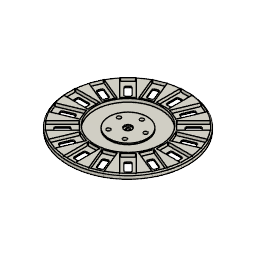
Brodie Rotor (Autodesk Fusion 360 design; units mm, degrees)
Autodesk Fusion 360 part; units mm, degrees
sketch "Sketch1" plane through (0, 0, 0) normal (0, 0, 1) x (1, 0, 0)
  circle A0 centre (0, 0) radius 26
  line L0 (-4.2, 27) -> (4.2, 27)
  line L1 (4.5, 27.3) -> (4.5, 45.7)
  line L2 (4.2, 46) -> (-4.2, 46)
  line L3 (-4.5, 45.7) -> (-4.5, 27.3)
  circle A1 centre (0, 0) radius 47
  line L4 (-4.5, 36.5) -> (4.5, 36.5) construction
  arc A2 (4.2, 27) -> (4.5, 27.3) centre (4.5, 27) ccw
  arc A3 (-4.5, 27.3) -> (-4.2, 27) centre (-4.5, 27) ccw
  arc A4 (-4.2, 46) -> (-4.5, 45.7) centre (-4.5, 46) ccw
  arc A5 (4.5, 45.7) -> (4.2, 46) centre (4.5, 46) ccw
  arc A6 (-13.3312, 43.9434) -> (-13.7231, 44.1057) centre (-13.446, 44.2205) ccw
  line L5 (-6.2898, 26.944) -> (-13.3312, 43.9434)
  line L6 (-13.7231, 44.1057) -> (-21.4837, 40.8912)
  arc A7 (-21.4837, 40.8912) -> (-21.6461, 40.4992) centre (-21.7609, 40.7764) ccw
  line L7 (-21.6461, 40.4992) -> (-14.6047, 23.4998)
  arc A8 (-14.6047, 23.4998) -> (-14.2127, 23.3375) centre (-14.4899, 23.2227) ccw
  line L8 (-14.2127, 23.3375) -> (-6.4522, 26.552)
  arc A9 (-6.4522, 26.552) -> (-6.2898, 26.944) centre (-6.175, 26.6668) ccw
  arc A10 (-29.1328, 35.4968) -> (-29.5571, 35.4968) centre (-29.3449, 35.7089) ccw
  line L9 (-16.122, 22.486) -> (-29.1328, 35.4968)
  line L10 (-29.5571, 35.4968) -> (-35.4968, 29.5571)
  arc A11 (-35.4968, 29.5571) -> (-35.4968, 29.1328) centre (-35.7089, 29.3449) ccw
  line L11 (-35.4968, 29.1328) -> (-22.486, 16.122)
  arc A12 (-22.486, 16.122) -> (-22.0617, 16.122) centre (-22.2739, 15.9099) ccw
  line L12 (-22.0617, 16.122) -> (-16.122, 22.0617)
  arc A13 (-16.122, 22.0617) -> (-16.122, 22.486) centre (-15.9099, 22.2739) ccw
  arc A14 (-40.4992, 21.6461) -> (-40.8912, 21.4837) centre (-40.7764, 21.7609) ccw
  line L13 (-23.4998, 14.6047) -> (-40.4992, 21.6461)
  line L14 (-40.8912, 21.4837) -> (-44.1057, 13.7231)
  arc A15 (-44.1057, 13.7231) -> (-43.9434, 13.3312) centre (-44.2205, 13.446) ccw
  line L15 (-43.9434, 13.3312) -> (-26.944, 6.2898)
  arc A16 (-26.944, 6.2898) -> (-26.552, 6.4522) centre (-26.6668, 6.175) ccw
  line L16 (-26.552, 6.4522) -> (-23.3375, 14.2127)
  arc A17 (-23.3375, 14.2127) -> (-23.4998, 14.6047) centre (-23.2227, 14.4899) ccw
  arc A18 (-45.7, 4.5) -> (-46, 4.2) centre (-46, 4.5) ccw
  line L17 (-27.3, 4.5) -> (-45.7, 4.5)
  line L18 (-46, 4.2) -> (-46, -4.2)
  arc A19 (-46, -4.2) -> (-45.7, -4.5) centre (-46, -4.5) ccw
  line L19 (-45.7, -4.5) -> (-27.3, -4.5)
  arc A20 (-27.3, -4.5) -> (-27, -4.2) centre (-27, -4.5) ccw
  line L20 (-27, -4.2) -> (-27, 4.2)
  arc A21 (-27, 4.2) -> (-27.3, 4.5) centre (-27, 4.5) ccw
  arc A22 (-43.9434, -13.3312) -> (-44.1057, -13.7231) centre (-44.2205, -13.446) ccw
  line L21 (-26.944, -6.2898) -> (-43.9434, -13.3312)
  line L22 (-44.1057, -13.7231) -> (-40.8912, -21.4837)
  arc A23 (-40.8912, -21.4837) -> (-40.4992, -21.6461) centre (-40.7764, -21.7609) ccw
  line L23 (-40.4992, -21.6461) -> (-23.4998, -14.6047)
  arc A24 (-23.4998, -14.6047) -> (-23.3375, -14.2127) centre (-23.2227, -14.4899) ccw
  line L24 (-23.3375, -14.2127) -> (-26.552, -6.4522)
  arc A25 (-26.552, -6.4522) -> (-26.944, -6.2898) centre (-26.6668, -6.175) ccw
  arc A26 (-35.4968, -29.1328) -> (-35.4968, -29.5571) centre (-35.7089, -29.3449) ccw
  line L25 (-22.486, -16.122) -> (-35.4968, -29.1328)
  line L26 (-35.4968, -29.5571) -> (-29.5571, -35.4968)
  arc A27 (-29.5571, -35.4968) -> (-29.1328, -35.4968) centre (-29.3449, -35.7089) ccw
  line L27 (-29.1328, -35.4968) -> (-16.122, -22.486)
  arc A28 (-16.122, -22.486) -> (-16.122, -22.0617) centre (-15.9099, -22.2739) ccw
  line L28 (-16.122, -22.0617) -> (-22.0617, -16.122)
  arc A29 (-22.0617, -16.122) -> (-22.486, -16.122) centre (-22.2739, -15.9099) ccw
  arc A30 (-21.6461, -40.4992) -> (-21.4837, -40.8912) centre (-21.7609, -40.7764) ccw
  line L29 (-14.6047, -23.4998) -> (-21.6461, -40.4992)
  line L30 (-21.4837, -40.8912) -> (-13.7231, -44.1057)
  arc A31 (-13.7231, -44.1057) -> (-13.3312, -43.9434) centre (-13.446, -44.2205) ccw
  line L31 (-13.3312, -43.9434) -> (-6.2898, -26.944)
  arc A32 (-6.2898, -26.944) -> (-6.4522, -26.552) centre (-6.175, -26.6668) ccw
  line L32 (-6.4522, -26.552) -> (-14.2127, -23.3375)
  arc A33 (-14.2127, -23.3375) -> (-14.6047, -23.4998) centre (-14.4899, -23.2227) ccw
  arc A34 (-4.5, -45.7) -> (-4.2, -46) centre (-4.5, -46) ccw
  line L33 (-4.5, -27.3) -> (-4.5, -45.7)
  line L34 (-4.2, -46) -> (4.2, -46)
  arc A35 (4.2, -46) -> (4.5, -45.7) centre (4.5, -46) ccw
  line L35 (4.5, -45.7) -> (4.5, -27.3)
  arc A36 (4.5, -27.3) -> (4.2, -27) centre (4.5, -27) ccw
  line L36 (4.2, -27) -> (-4.2, -27)
  arc A37 (-4.2, -27) -> (-4.5, -27.3) centre (-4.5, -27) ccw
  arc A38 (13.3312, -43.9434) -> (13.7231, -44.1057) centre (13.446, -44.2205) ccw
  line L37 (6.2898, -26.944) -> (13.3312, -43.9434)
  line L38 (13.7231, -44.1057) -> (21.4837, -40.8912)
  arc A39 (21.4837, -40.8912) -> (21.6461, -40.4992) centre (21.7609, -40.7764) ccw
  line L39 (21.6461, -40.4992) -> (14.6047, -23.4998)
  arc A40 (14.6047, -23.4998) -> (14.2127, -23.3375) centre (14.4899, -23.2227) ccw
  line L40 (14.2127, -23.3375) -> (6.4522, -26.552)
  arc A41 (6.4522, -26.552) -> (6.2898, -26.944) centre (6.175, -26.6668) ccw
  arc A42 (29.1328, -35.4968) -> (29.5571, -35.4968) centre (29.3449, -35.7089) ccw
  line L41 (16.122, -22.486) -> (29.1328, -35.4968)
  line L42 (29.5571, -35.4968) -> (35.4968, -29.5571)
  arc A43 (35.4968, -29.5571) -> (35.4968, -29.1328) centre (35.7089, -29.3449) ccw
  line L43 (35.4968, -29.1328) -> (22.486, -16.122)
  arc A44 (22.486, -16.122) -> (22.0617, -16.122) centre (22.2739, -15.9099) ccw
  line L44 (22.0617, -16.122) -> (16.122, -22.0617)
  arc A45 (16.122, -22.0617) -> (16.122, -22.486) centre (15.9099, -22.2739) ccw
  arc A46 (40.4992, -21.6461) -> (40.8912, -21.4837) centre (40.7764, -21.7609) ccw
  line L45 (23.4998, -14.6047) -> (40.4992, -21.6461)
  line L46 (40.8912, -21.4837) -> (44.1057, -13.7231)
  arc A47 (44.1057, -13.7231) -> (43.9434, -13.3312) centre (44.2205, -13.446) ccw
  line L47 (43.9434, -13.3312) -> (26.944, -6.2898)
  arc A48 (26.944, -6.2898) -> (26.552, -6.4522) centre (26.6668, -6.175) ccw
  line L48 (26.552, -6.4522) -> (23.3375, -14.2127)
  arc A49 (23.3375, -14.2127) -> (23.4998, -14.6047) centre (23.2227, -14.4899) ccw
  arc A50 (45.7, -4.5) -> (46, -4.2) centre (46, -4.5) ccw
  line L49 (27.3, -4.5) -> (45.7, -4.5)
  line L50 (46, -4.2) -> (46, 4.2)
  arc A51 (46, 4.2) -> (45.7, 4.5) centre (46, 4.5) ccw
  line L51 (45.7, 4.5) -> (27.3, 4.5)
  arc A52 (27.3, 4.5) -> (27, 4.2) centre (27, 4.5) ccw
  line L52 (27, 4.2) -> (27, -4.2)
  arc A53 (27, -4.2) -> (27.3, -4.5) centre (27, -4.5) ccw
  arc A54 (43.9434, 13.3312) -> (44.1057, 13.7231) centre (44.2205, 13.446) ccw
  line L53 (26.944, 6.2898) -> (43.9434, 13.3312)
  line L54 (44.1057, 13.7231) -> (40.8912, 21.4837)
  arc A55 (40.8912, 21.4837) -> (40.4992, 21.6461) centre (40.7764, 21.7609) ccw
  line L55 (40.4992, 21.6461) -> (23.4998, 14.6047)
  arc A56 (23.4998, 14.6047) -> (23.3375, 14.2127) centre (23.2227, 14.4899) ccw
  line L56 (23.3375, 14.2127) -> (26.552, 6.4522)
  arc A57 (26.552, 6.4522) -> (26.944, 6.2898) centre (26.6668, 6.175) ccw
  arc A58 (35.4968, 29.1328) -> (35.4968, 29.5571) centre (35.7089, 29.3449) ccw
  line L57 (22.486, 16.122) -> (35.4968, 29.1328)
  line L58 (35.4968, 29.5571) -> (29.5571, 35.4968)
  arc A59 (29.5571, 35.4968) -> (29.1328, 35.4968) centre (29.3449, 35.7089) ccw
  line L59 (29.1328, 35.4968) -> (16.122, 22.486)
  arc A60 (16.122, 22.486) -> (16.122, 22.0617) centre (15.9099, 22.2739) ccw
  line L60 (16.122, 22.0617) -> (22.0617, 16.122)
  arc A61 (22.0617, 16.122) -> (22.486, 16.122) centre (22.2739, 15.9099) ccw
  arc A62 (21.6461, 40.4992) -> (21.4837, 40.8912) centre (21.7609, 40.7764) ccw
  line L61 (14.6047, 23.4998) -> (21.6461, 40.4992)
  line L62 (21.4837, 40.8912) -> (13.7231, 44.1057)
  arc A63 (13.7231, 44.1057) -> (13.3312, 43.9434) centre (13.446, 44.2205) ccw
  line L63 (13.3312, 43.9434) -> (6.2898, 26.944)
  arc A64 (6.2898, 26.944) -> (6.4522, 26.552) centre (6.175, 26.6668) ccw
  line L64 (6.4522, 26.552) -> (14.2127, 23.3375)
  arc A65 (14.2127, 23.3375) -> (14.6047, 23.4998) centre (14.4899, 23.2227) ccw
  dimension "d1" = 52
  dimension "d6" = 94
  dimension "d7" = 0.6
  dimension "d8" = 0.6
  dimension "d10" = 360
  constraint coincident A0.centre A1.centre
  constraint horizontal L0
  constraint vertical L1
  constraint horizontal L2
  constraint vertical L3
  constraint concentric A0 A1
  constraint symmetric L4 A3 A4
  constraint symmetric L4 A2 A5
  constraint coincident L1 L4.end
  constraint coincident L3 L4.start
  measures "d1" diameter of A0
  measures "d6" diameter of A1
  measures "d7" diameter of A4
  measures "d8" diameter of A5
extrude "Extrude1" add sketch "Sketch1" along normal blind 2.5
sketch "Sketch2" plane through (0, 0, 0) normal (0, 0, 1) x (1, 0, 0)
  circle A0 centre (0, 0) radius 47
  dimension "d13" = 94
  constraint coincident A0.centre origin
  measures "d13" diameter of A0
extrude "Extrude2" add sketch "Sketch2" against normal blind 1
move_body "Move1" bodies 1 to x (1, 0, 0) y (0, 1, 0) z (0, 0, 1) at (0, 0, 1)
sketch "Sketch3" plane through (0, 0, 1) normal (0, 0, 1) x (-1, 0, 0)
  circle A0 centre (0, 0) radius 26
  circle A1 centre (0, 0) radius 15
  dimension "d16" = 30
  constraint coincident A0.centre A1.centre
  measures "d16" diameter of A1
extrude "Extrude3" add sketch "Sketch3" along normal blind 1 contours A1
sketch "Sketch4" plane through (0, 0, 2) normal (0, 0, 1) x (-1, 0, 0)
  circle A0 centre (0, 0) radius 15
  circle A1 centre (0, 0) radius 3
  circle A2 centre (0, -11) radius 1.5
  circle A3 centre (10.4616, -3.3992) radius 1.5
  circle A4 centre (6.4656, 8.8992) radius 1.5
  circle A5 centre (-6.4656, 8.8992) radius 1.5
  circle A6 centre (-10.4616, -3.3992) radius 1.5
  dimension "d19" = 3
  dimension "d21" = 360
  constraint coincident A0.centre A1.centre
  measures "d19" diameter of A2
extrude "Extrude4" cut sketch "Sketch4" against normal blind 10 contours A2 | A3 | A4 | A5 | A6
extrude "Extrude5" add sketch "Sketch4" along normal blind 1 contours A1
sketch "Sketch5" plane through (0, 0, 3) normal (0, 0, 1) x (-1, 0, 0)
  circle A0 centre (0, 0) radius 3
  circle A1 centre (0, 0) radius 1.5
  dimension "d26" = 3
  constraint coincident A0.centre A1.centre
  measures "d26" diameter of A1
extrude "Extrude6" cut sketch "Sketch5" against normal blind 10 contours A1
extrude "Extrude7" cut 1 faces at (-2.4832, 0.2236, 3) along direction (0, 0, -1) blind 2
sketch "Sketch6" plane through (0, 0, 0) normal (0, 0, -1) x (1, 0, 0)
  circle A0 centre (0, 0) radius 1.5
  circle A1 centre (-6.4656, 8.8992) radius 1.5
  circle A2 centre (-10.4616, -3.3992) radius 1.5
  circle A3 centre (6.4656, 8.8992) radius 1.5
  circle A4 centre (0, -11) radius 1.5
  circle A5 centre (10.4616, -3.3992) radius 1.5
  circle A6 centre (0, 0) radius 47
  line L0 (-1.25, -31.75) -> (1.25, -31.75)
  line L1 (2.25, -32.75) -> (2.25, -40.25)
  line L2 (1.25, -41.25) -> (-1.25, -41.25)
  line L3 (-2.25, -40.25) -> (-2.25, -32.75)
  arc A7 (1.25, -41.25) -> (2.25, -40.25) centre (1.25, -40.25) ccw
  arc A8 (-2.25, -40.25) -> (-1.25, -41.25) centre (-1.25, -40.25) ccw
  arc A9 (-1.25, -31.75) -> (-2.25, -32.75) centre (-1.25, -32.75) ccw
  arc A10 (2.25, -32.75) -> (1.25, -31.75) centre (1.25, -32.75) ccw
  line L4 (2.25, -31.75) -> (2.0564, -32.1587) construction
  line L5 (-2.0564, -40.8413) -> (-2.25, -41.25) construction
  line L6 (-2.25, -31.75) -> (-2.0564, -32.1587) construction
  line L7 (2.0564, -40.8413) -> (2.25, -41.25) construction
  line L8 (13.3243, -38.0472) -> (10.4542, -31.1181)
  arc A11 (10.9953, -29.8115) -> (10.4542, -31.1181) centre (11.378, -30.7354) ccw
  arc A12 (14.6116, -29.396) -> (13.305, -28.8548) centre (13.6877, -29.7787) ccw
  line L9 (10.9953, -29.8115) -> (13.305, -28.8548)
  line L10 (14.6116, -29.396) -> (17.4817, -36.3251)
  arc A13 (16.9405, -37.6317) -> (17.4817, -36.3251) centre (16.5579, -36.7078) ccw
  line L11 (16.9405, -37.6317) -> (14.6308, -38.5884)
  arc A14 (13.3243, -38.0472) -> (14.6308, -38.5884) centre (14.2482, -37.6645) ccw
  line L12 (26.8701, -30.052) -> (21.5668, -24.7487)
  arc A15 (21.5668, -23.3345) -> (21.5668, -24.7487) centre (22.2739, -24.0416) ccw
  arc A16 (24.7487, -21.5668) -> (23.3345, -21.5668) centre (24.0416, -22.2739) ccw
  line L13 (21.5668, -23.3345) -> (23.3345, -21.5668)
  line L14 (24.7487, -21.5668) -> (30.052, -26.8701)
  arc A17 (30.052, -28.2843) -> (30.052, -26.8701) centre (29.3449, -27.5772) ccw
  line L15 (30.052, -28.2843) -> (28.2843, -30.052)
  arc A18 (26.8701, -30.052) -> (28.2843, -30.052) centre (27.5772, -29.3449) ccw
  line L16 (36.3251, -17.4817) -> (29.396, -14.6116)
  arc A19 (28.8548, -13.305) -> (29.396, -14.6116) centre (29.7787, -13.6877) ccw
  arc A20 (31.1181, -10.4542) -> (29.8115, -10.9953) centre (30.7354, -11.378) ccw
  line L17 (28.8548, -13.305) -> (29.8115, -10.9953)
  line L18 (31.1181, -10.4542) -> (38.0472, -13.3243)
  arc A21 (38.5884, -14.6308) -> (38.0472, -13.3243) centre (37.6645, -14.2482) ccw
  line L19 (38.5884, -14.6308) -> (37.6317, -16.9405)
  arc A22 (36.3251, -17.4817) -> (37.6317, -16.9405) centre (36.7078, -16.5579) ccw
  line L20 (40.25, -2.25) -> (32.75, -2.25)
  arc A23 (31.75, -1.25) -> (32.75, -2.25) centre (32.75, -1.25) ccw
  arc A24 (32.75, 2.25) -> (31.75, 1.25) centre (32.75, 1.25) ccw
  line L21 (31.75, -1.25) -> (31.75, 1.25)
  line L22 (32.75, 2.25) -> (40.25, 2.25)
  arc A25 (41.25, 1.25) -> (40.25, 2.25) centre (40.25, 1.25) ccw
  line L23 (41.25, 1.25) -> (41.25, -1.25)
  arc A26 (40.25, -2.25) -> (41.25, -1.25) centre (40.25, -1.25) ccw
  line L24 (38.0472, 13.3243) -> (31.1181, 10.4542)
  arc A27 (29.8115, 10.9953) -> (31.1181, 10.4542) centre (30.7354, 11.378) ccw
  arc A28 (29.396, 14.6116) -> (28.8548, 13.305) centre (29.7787, 13.6877) ccw
  line L25 (29.8115, 10.9953) -> (28.8548, 13.305)
  line L26 (29.396, 14.6116) -> (36.3251, 17.4817)
  arc A29 (37.6317, 16.9405) -> (36.3251, 17.4817) centre (36.7078, 16.5579) ccw
  line L27 (37.6317, 16.9405) -> (38.5884, 14.6308)
  arc A30 (38.0472, 13.3243) -> (38.5884, 14.6308) centre (37.6645, 14.2482) ccw
  line L28 (30.052, 26.8701) -> (24.7487, 21.5668)
  arc A31 (23.3345, 21.5668) -> (24.7487, 21.5668) centre (24.0416, 22.2739) ccw
  arc A32 (21.5668, 24.7487) -> (21.5668, 23.3345) centre (22.2739, 24.0416) ccw
  line L29 (23.3345, 21.5668) -> (21.5668, 23.3345)
  line L30 (21.5668, 24.7487) -> (26.8701, 30.052)
  arc A33 (28.2843, 30.052) -> (26.8701, 30.052) centre (27.5772, 29.3449) ccw
  line L31 (28.2843, 30.052) -> (30.052, 28.2843)
  arc A34 (30.052, 26.8701) -> (30.052, 28.2843) centre (29.3449, 27.5772) ccw
  line L32 (17.4817, 36.3251) -> (14.6116, 29.396)
  arc A35 (13.305, 28.8548) -> (14.6116, 29.396) centre (13.6877, 29.7787) ccw
  arc A36 (10.4542, 31.1181) -> (10.9953, 29.8115) centre (11.378, 30.7354) ccw
  line L33 (13.305, 28.8548) -> (10.9953, 29.8115)
  line L34 (10.4542, 31.1181) -> (13.3243, 38.0472)
  arc A37 (14.6308, 38.5884) -> (13.3243, 38.0472) centre (14.2482, 37.6645) ccw
  line L35 (14.6308, 38.5884) -> (16.9405, 37.6317)
  arc A38 (17.4817, 36.3251) -> (16.9405, 37.6317) centre (16.5579, 36.7078) ccw
  line L36 (2.25, 40.25) -> (2.25, 32.75)
  arc A39 (1.25, 31.75) -> (2.25, 32.75) centre (1.25, 32.75) ccw
  arc A40 (-2.25, 32.75) -> (-1.25, 31.75) centre (-1.25, 32.75) ccw
  line L37 (1.25, 31.75) -> (-1.25, 31.75)
  line L38 (-2.25, 32.75) -> (-2.25, 40.25)
  arc A41 (-1.25, 41.25) -> (-2.25, 40.25) centre (-1.25, 40.25) ccw
  line L39 (-1.25, 41.25) -> (1.25, 41.25)
  arc A42 (2.25, 40.25) -> (1.25, 41.25) centre (1.25, 40.25) ccw
  line L40 (-13.3243, 38.0472) -> (-10.4542, 31.1181)
  arc A43 (-10.9953, 29.8115) -> (-10.4542, 31.1181) centre (-11.378, 30.7354) ccw
  arc A44 (-14.6116, 29.396) -> (-13.305, 28.8548) centre (-13.6877, 29.7787) ccw
  line L41 (-10.9953, 29.8115) -> (-13.305, 28.8548)
  line L42 (-14.6116, 29.396) -> (-17.4817, 36.3251)
  arc A45 (-16.9405, 37.6317) -> (-17.4817, 36.3251) centre (-16.5579, 36.7078) ccw
  line L43 (-16.9405, 37.6317) -> (-14.6308, 38.5884)
  arc A46 (-13.3243, 38.0472) -> (-14.6308, 38.5884) centre (-14.2482, 37.6645) ccw
  line L44 (-26.8701, 30.052) -> (-21.5668, 24.7487)
  arc A47 (-21.5668, 23.3345) -> (-21.5668, 24.7487) centre (-22.2739, 24.0416) ccw
  arc A48 (-24.7487, 21.5668) -> (-23.3345, 21.5668) centre (-24.0416, 22.2739) ccw
  line L45 (-21.5668, 23.3345) -> (-23.3345, 21.5668)
  line L46 (-24.7487, 21.5668) -> (-30.052, 26.8701)
  arc A49 (-30.052, 28.2843) -> (-30.052, 26.8701) centre (-29.3449, 27.5772) ccw
  line L47 (-30.052, 28.2843) -> (-28.2843, 30.052)
  arc A50 (-26.8701, 30.052) -> (-28.2843, 30.052) centre (-27.5772, 29.3449) ccw
  line L48 (-36.3251, 17.4817) -> (-29.396, 14.6116)
  arc A51 (-28.8548, 13.305) -> (-29.396, 14.6116) centre (-29.7787, 13.6877) ccw
  arc A52 (-31.1181, 10.4542) -> (-29.8115, 10.9953) centre (-30.7354, 11.378) ccw
  line L49 (-28.8548, 13.305) -> (-29.8115, 10.9953)
  line L50 (-31.1181, 10.4542) -> (-38.0472, 13.3243)
  arc A53 (-38.5884, 14.6308) -> (-38.0472, 13.3243) centre (-37.6645, 14.2482) ccw
  line L51 (-38.5884, 14.6308) -> (-37.6317, 16.9405)
  arc A54 (-36.3251, 17.4817) -> (-37.6317, 16.9405) centre (-36.7078, 16.5579) ccw
  line L52 (-40.25, 2.25) -> (-32.75, 2.25)
  arc A55 (-31.75, 1.25) -> (-32.75, 2.25) centre (-32.75, 1.25) ccw
  arc A56 (-32.75, -2.25) -> (-31.75, -1.25) centre (-32.75, -1.25) ccw
  line L53 (-31.75, 1.25) -> (-31.75, -1.25)
  line L54 (-32.75, -2.25) -> (-40.25, -2.25)
  arc A57 (-41.25, -1.25) -> (-40.25, -2.25) centre (-40.25, -1.25) ccw
  line L55 (-41.25, -1.25) -> (-41.25, 1.25)
  arc A58 (-40.25, 2.25) -> (-41.25, 1.25) centre (-40.25, 1.25) ccw
  line L56 (-38.0472, -13.3243) -> (-31.1181, -10.4542)
  arc A59 (-29.8115, -10.9953) -> (-31.1181, -10.4542) centre (-30.7354, -11.378) ccw
  arc A60 (-29.396, -14.6116) -> (-28.8548, -13.305) centre (-29.7787, -13.6877) ccw
  line L57 (-29.8115, -10.9953) -> (-28.8548, -13.305)
  line L58 (-29.396, -14.6116) -> (-36.3251, -17.4817)
  arc A61 (-37.6317, -16.9405) -> (-36.3251, -17.4817) centre (-36.7078, -16.5579) ccw
  line L59 (-37.6317, -16.9405) -> (-38.5884, -14.6308)
  arc A62 (-38.0472, -13.3243) -> (-38.5884, -14.6308) centre (-37.6645, -14.2482) ccw
  line L60 (-30.052, -26.8701) -> (-24.7487, -21.5668)
  arc A63 (-23.3345, -21.5668) -> (-24.7487, -21.5668) centre (-24.0416, -22.2739) ccw
  arc A64 (-21.5668, -24.7487) -> (-21.5668, -23.3345) centre (-22.2739, -24.0416) ccw
  line L61 (-23.3345, -21.5668) -> (-21.5668, -23.3345)
  line L62 (-21.5668, -24.7487) -> (-26.8701, -30.052)
  arc A65 (-28.2843, -30.052) -> (-26.8701, -30.052) centre (-27.5772, -29.3449) ccw
  line L63 (-28.2843, -30.052) -> (-30.052, -28.2843)
  arc A66 (-30.052, -26.8701) -> (-30.052, -28.2843) centre (-29.3449, -27.5772) ccw
  line L64 (-17.4817, -36.3251) -> (-14.6116, -29.396)
  arc A67 (-13.305, -28.8548) -> (-14.6116, -29.396) centre (-13.6877, -29.7787) ccw
  arc A68 (-10.4542, -31.1181) -> (-10.9953, -29.8115) centre (-11.378, -30.7354) ccw
  line L65 (-13.305, -28.8548) -> (-10.9953, -29.8115)
  line L66 (-10.4542, -31.1181) -> (-13.3243, -38.0472)
  arc A69 (-14.6308, -38.5884) -> (-13.3243, -38.0472) centre (-14.2482, -37.6645) ccw
  line L67 (-14.6308, -38.5884) -> (-16.9405, -37.6317)
  arc A70 (-17.4817, -36.3251) -> (-16.9405, -37.6317) centre (-16.5579, -36.7078) ccw
  dimension "d32" = 4.5
  dimension "d33" = 9.5
  dimension "d34" = 1
  dimension "d36" = 360
  constraint horizontal L0
  constraint perpendicular L0 L1
  constraint parallel L0 L2
  constraint parallel L1 L3
  constraint coincident L7.end L2
  constraint coincident L7.end L1
  constraint tangent L2 A7
  constraint tangent L1 A7
  constraint coincident L5.end L2
  constraint coincident L5.end L3
  constraint tangent L2 A8
  constraint tangent L3 A8
  constraint equal A7 A8
  constraint coincident L6.start L3
  constraint coincident L6.start L0
  constraint tangent L3 A9
  constraint tangent L0 A9
  constraint equal A7 A9
  constraint coincident L4.start L0
  constraint coincident L4.start L1
  constraint tangent L0 A10
  constraint tangent L1 A10
  constraint equal A7 A10
  constraint coincident A8 L5.start
  constraint collinear L4 L5
  constraint coincident A7 L7.start
  constraint collinear L6 L7
  constraint coincident A10 L4.end
  constraint coincident A9 L6.end
  measures "d32" distance of L7.end L5.end
  measures "d33" distance of L4.start L7.end
  measures "d34" radius of A7
extrude "Extrude8" cut sketch "Sketch6" against normal blind 10 contours L0 L1 L2 L3 A7 A8 A9 A10 | L8 A11 A12 L9 L10 A13 L11 A14 | L12 A15 A16 L13 L14 A17 L15 A18 | L16 A19 A20 L17 L18 A21 L19 A22 | L20 A23 A24 L21 L22 A25 L23 A26 | L24 A27 A28 L25 L26 A29 L27 A30 | L28 A31 A32 L29 L30 A33 L31 A34 | L32 A35 A36 L33 L34 A37 L35 A38 | L36 A39 A40 L37 L38 A41 L39 A42 | L40 A43 A44 L41 L42 A45 L43 A46 | L44 A47 A48 L45 L46 A49 L47 A50 | L48 A51 A52 L49 L50 A53 L51 A54 | L52 A55 A56 L53 L54 A57 L55 A58 | L56 A59 A60 L57 L58 A61 L59 A62 | L60 A63 A64 L61 L62 A65 L63 A66 | L64 A67 A68 L65 L66 A69 L67 A70
fillet "Fillet1" radius 1 1 edges at (-43.8194, -16.9959, 3.5)
extrude "Extrude9" cut 1 faces at (10.559, -3.3616, 2) along direction (0, 0, -1) blind 0.5
extrude "Extrude10" add 1 faces at (10.559, -3.3616, 1.5) along direction (0, 0, 1) blind 0.5
sketch "Sketch7" plane through (0, 0, 3.5) normal (0, 0, 1) x (-1, 0, 0)
  circle A0 centre (0, 0) radius 26
  arc A1 (13.1869, 44.0693) -> (4.6815, 45.7612) centre (0, 0) ccw
  arc A2 (4.5, 45.7) -> (4.6815, 45.7612) centre (4.5, 46) ccw
  line L0 (4.5, 45.7) -> (4.5, 27.3)
  arc A3 (4.2, 27) -> (4.5, 27.3) centre (4.5, 27) ccw
  line L1 (4.2, 27) -> (-4.2, 27)
  arc A4 (-4.5, 27.3) -> (-4.2, 27) centre (-4.5, 27) ccw
  line L2 (-4.5, 27.3) -> (-4.5, 45.7)
  arc A5 (-4.6815, 45.7612) -> (-4.5, 45.7) centre (-4.5, 46) ccw
  arc A6 (-4.6815, 45.7612) -> (-13.1869, 44.0693) centre (0, 0) ccw
  arc A7 (-13.3312, 43.9434) -> (-13.1869, 44.0693) centre (-13.446, 44.2205) ccw
  line L3 (-13.3312, 43.9434) -> (-6.2898, 26.944)
  arc A8 (-6.4522, 26.552) -> (-6.2898, 26.944) centre (-6.175, 26.6668) ccw
  line L4 (-6.4522, 26.552) -> (-14.2127, 23.3375)
  arc A9 (-14.6047, 23.4998) -> (-14.2127, 23.3375) centre (-14.4899, 23.2227) ccw
  line L5 (-14.6047, 23.4998) -> (-21.6461, 40.4992)
  arc A10 (-21.8372, 40.4863) -> (-21.6461, 40.4992) centre (-21.7609, 40.7764) ccw
  arc A11 (-21.8372, 40.4863) -> (-29.0477, 35.6684) centre (0, 0) ccw
  arc A12 (-29.1328, 35.4968) -> (-29.0477, 35.6684) centre (-29.3449, 35.7089) ccw
  line L6 (-29.1328, 35.4968) -> (-16.122, 22.486)
  arc A13 (-16.122, 22.0617) -> (-16.122, 22.486) centre (-15.9099, 22.2739) ccw
  line L7 (-16.122, 22.0617) -> (-22.0617, 16.122)
  arc A14 (-22.486, 16.122) -> (-22.0617, 16.122) centre (-22.2739, 15.9099) ccw
  line L8 (-22.486, 16.122) -> (-35.4968, 29.1328)
  arc A15 (-35.6684, 29.0477) -> (-35.4968, 29.1328) centre (-35.7089, 29.3449) ccw
  arc A16 (-35.6684, 29.0477) -> (-40.4863, 21.8372) centre (0, 0) ccw
  arc A17 (-40.4992, 21.6461) -> (-40.4863, 21.8372) centre (-40.7764, 21.7609) ccw
  line L9 (-40.4992, 21.6461) -> (-23.4998, 14.6047)
  arc A18 (-23.3375, 14.2127) -> (-23.4998, 14.6047) centre (-23.2227, 14.4899) ccw
  line L10 (-23.3375, 14.2127) -> (-26.552, 6.4522)
  arc A19 (-26.944, 6.2898) -> (-26.552, 6.4522) centre (-26.6668, 6.175) ccw
  line L11 (-26.944, 6.2898) -> (-43.9434, 13.3312)
  arc A20 (-44.0693, 13.1869) -> (-43.9434, 13.3312) centre (-44.2205, 13.446) ccw
  arc A21 (-44.0693, 13.1869) -> (-45.7612, 4.6815) centre (0, 0) ccw
  arc A22 (-45.7, 4.5) -> (-45.7612, 4.6815) centre (-46, 4.5) ccw
  line L12 (-45.7, 4.5) -> (-27.3, 4.5)
  arc A23 (-27, 4.2) -> (-27.3, 4.5) centre (-27, 4.5) ccw
  line L13 (-27, 4.2) -> (-27, -4.2)
  arc A24 (-27.3, -4.5) -> (-27, -4.2) centre (-27, -4.5) ccw
  line L14 (-27.3, -4.5) -> (-45.7, -4.5)
  arc A25 (-45.7612, -4.6815) -> (-45.7, -4.5) centre (-46, -4.5) ccw
  arc A26 (-45.7612, -4.6815) -> (-44.0693, -13.1869) centre (0, 0) ccw
  arc A27 (-43.9434, -13.3312) -> (-44.0693, -13.1869) centre (-44.2205, -13.446) ccw
  line L15 (-43.9434, -13.3312) -> (-26.944, -6.2898)
  arc A28 (-26.552, -6.4522) -> (-26.944, -6.2898) centre (-26.6668, -6.175) ccw
  line L16 (-26.552, -6.4522) -> (-23.3375, -14.2127)
  arc A29 (-23.4998, -14.6047) -> (-23.3375, -14.2127) centre (-23.2227, -14.4899) ccw
  line L17 (-23.4998, -14.6047) -> (-40.4992, -21.6461)
  arc A30 (-40.4863, -21.8372) -> (-40.4992, -21.6461) centre (-40.7764, -21.7609) ccw
  arc A31 (-40.4863, -21.8372) -> (-35.6684, -29.0477) centre (0, 0) ccw
  arc A32 (-35.4968, -29.1328) -> (-35.6684, -29.0477) centre (-35.7089, -29.3449) ccw
  line L18 (-35.4968, -29.1328) -> (-22.486, -16.122)
  arc A33 (-22.0617, -16.122) -> (-22.486, -16.122) centre (-22.2739, -15.9099) ccw
  line L19 (-22.0617, -16.122) -> (-16.122, -22.0617)
  arc A34 (-16.122, -22.486) -> (-16.122, -22.0617) centre (-15.9099, -22.2739) ccw
  line L20 (-16.122, -22.486) -> (-29.1328, -35.4968)
  arc A35 (-29.0477, -35.6684) -> (-29.1328, -35.4968) centre (-29.3449, -35.7089) ccw
  arc A36 (-29.0477, -35.6684) -> (-21.8372, -40.4863) centre (0, 0) ccw
  arc A37 (-21.6461, -40.4992) -> (-21.8372, -40.4863) centre (-21.7609, -40.7764) ccw
  line L21 (-21.6461, -40.4992) -> (-14.6047, -23.4998)
  arc A38 (-14.2127, -23.3375) -> (-14.6047, -23.4998) centre (-14.4899, -23.2227) ccw
  line L22 (-14.2127, -23.3375) -> (-6.4522, -26.552)
  arc A39 (-6.2898, -26.944) -> (-6.4522, -26.552) centre (-6.175, -26.6668) ccw
  line L23 (-6.2898, -26.944) -> (-13.3312, -43.9434)
  arc A40 (-13.1869, -44.0693) -> (-13.3312, -43.9434) centre (-13.446, -44.2205) ccw
  arc A41 (-13.1869, -44.0693) -> (-4.6815, -45.7612) centre (0, 0) ccw
  arc A42 (-4.5, -45.7) -> (-4.6815, -45.7612) centre (-4.5, -46) ccw
  line L24 (-4.5, -45.7) -> (-4.5, -27.3)
  arc A43 (-4.2, -27) -> (-4.5, -27.3) centre (-4.5, -27) ccw
  line L25 (-4.2, -27) -> (4.2, -27)
  arc A44 (4.5, -27.3) -> (4.2, -27) centre (4.5, -27) ccw
  line L26 (4.5, -27.3) -> (4.5, -45.7)
  arc A45 (4.6815, -45.7612) -> (4.5, -45.7) centre (4.5, -46) ccw
  arc A46 (4.6815, -45.7612) -> (13.1869, -44.0693) centre (0, 0) ccw
  arc A47 (13.3312, -43.9434) -> (13.1869, -44.0693) centre (13.446, -44.2205) ccw
  line L27 (13.3312, -43.9434) -> (6.2898, -26.944)
  arc A48 (6.4522, -26.552) -> (6.2898, -26.944) centre (6.175, -26.6668) ccw
  line L28 (6.4522, -26.552) -> (14.2127, -23.3375)
  arc A49 (14.6047, -23.4998) -> (14.2127, -23.3375) centre (14.4899, -23.2227) ccw
  line L29 (14.6047, -23.4998) -> (21.6461, -40.4992)
  arc A50 (21.8372, -40.4863) -> (21.6461, -40.4992) centre (21.7609, -40.7764) ccw
  arc A51 (21.8372, -40.4863) -> (29.0477, -35.6684) centre (0, 0) ccw
  arc A52 (29.1328, -35.4968) -> (29.0477, -35.6684) centre (29.3449, -35.7089) ccw
  line L30 (29.1328, -35.4968) -> (16.122, -22.486)
  arc A53 (16.122, -22.0617) -> (16.122, -22.486) centre (15.9099, -22.2739) ccw
  line L31 (16.122, -22.0617) -> (22.0617, -16.122)
  arc A54 (22.486, -16.122) -> (22.0617, -16.122) centre (22.2739, -15.9099) ccw
  line L32 (22.486, -16.122) -> (35.4968, -29.1328)
  arc A55 (35.6684, -29.0477) -> (35.4968, -29.1328) centre (35.7089, -29.3449) ccw
  arc A56 (35.6684, -29.0477) -> (40.4863, -21.8372) centre (0, 0) ccw
  arc A57 (40.4992, -21.6461) -> (40.4863, -21.8372) centre (40.7764, -21.7609) ccw
  line L33 (40.4992, -21.6461) -> (23.4998, -14.6047)
  arc A58 (23.3375, -14.2127) -> (23.4998, -14.6047) centre (23.2227, -14.4899) ccw
  line L34 (23.3375, -14.2127) -> (26.552, -6.4522)
  arc A59 (26.944, -6.2898) -> (26.552, -6.4522) centre (26.6668, -6.175) ccw
  line L35 (26.944, -6.2898) -> (43.9434, -13.3312)
  arc A60 (44.0693, -13.1869) -> (43.9434, -13.3312) centre (44.2205, -13.446) ccw
  arc A61 (44.0693, -13.1869) -> (45.7612, -4.6815) centre (0, 0) ccw
  arc A62 (45.7, -4.5) -> (45.7612, -4.6815) centre (46, -4.5) ccw
  line L36 (45.7, -4.5) -> (27.3, -4.5)
  arc A63 (27, -4.2) -> (27.3, -4.5) centre (27, -4.5) ccw
  line L37 (27, -4.2) -> (27, 4.2)
  arc A64 (27.3, 4.5) -> (27, 4.2) centre (27, 4.5) ccw
  line L38 (27.3, 4.5) -> (45.7, 4.5)
  arc A65 (45.7612, 4.6815) -> (45.7, 4.5) centre (46, 4.5) ccw
  arc A66 (45.7612, 4.6815) -> (44.0693, 13.1869) centre (0, 0) ccw
  arc A67 (43.9434, 13.3312) -> (44.0693, 13.1869) centre (44.2205, 13.446) ccw
  line L39 (43.9434, 13.3312) -> (26.944, 6.2898)
  arc A68 (26.552, 6.4522) -> (26.944, 6.2898) centre (26.6668, 6.175) ccw
  line L40 (26.552, 6.4522) -> (23.3375, 14.2127)
  arc A69 (23.4998, 14.6047) -> (23.3375, 14.2127) centre (23.2227, 14.4899) ccw
  line L41 (23.4998, 14.6047) -> (40.4992, 21.6461)
  arc A70 (40.4863, 21.8372) -> (40.4992, 21.6461) centre (40.7764, 21.7609) ccw
  arc A71 (40.4863, 21.8372) -> (35.6684, 29.0477) centre (0, 0) ccw
  arc A72 (35.4968, 29.1328) -> (35.6684, 29.0477) centre (35.7089, 29.3449) ccw
  line L42 (35.4968, 29.1328) -> (22.486, 16.122)
  arc A73 (22.0617, 16.122) -> (22.486, 16.122) centre (22.2739, 15.9099) ccw
  line L43 (22.0617, 16.122) -> (16.122, 22.0617)
  arc A74 (16.122, 22.486) -> (16.122, 22.0617) centre (15.9099, 22.2739) ccw
  line L44 (16.122, 22.486) -> (29.1328, 35.4968)
  arc A75 (29.0477, 35.6684) -> (29.1328, 35.4968) centre (29.3449, 35.7089) ccw
  arc A76 (29.0477, 35.6684) -> (21.8372, 40.4863) centre (0, 0) ccw
  arc A77 (21.6461, 40.4992) -> (21.8372, 40.4863) centre (21.7609, 40.7764) ccw
  line L45 (21.6461, 40.4992) -> (14.6047, 23.4998)
  arc A78 (14.2127, 23.3375) -> (14.6047, 23.4998) centre (14.4899, 23.2227) ccw
  line L46 (14.2127, 23.3375) -> (6.4522, 26.552)
  arc A79 (6.2898, 26.944) -> (6.4522, 26.552) centre (6.175, 26.6668) ccw
  line L47 (6.2898, 26.944) -> (13.3312, 43.9434)
  arc A80 (13.1869, 44.0693) -> (13.3312, 43.9434) centre (13.446, 44.2205) ccw
  line L48 (0, 0) -> (0, -37)
  line L49 (-4.6, -27) -> (4.6, -27)
  line L50 (4.6, -27) -> (4.6, -46)
  line L51 (4.6, -46) -> (-4.6, -46)
  line L52 (-4.6, -46) -> (-4.6, -27)
  line L53 (-4.6, -27) -> (4.6, -46) construction
  line L54 (4.6, -27) -> (-4.6, -46) construction
  line L55 (13.3536, -44.2588) -> (6.0826, -26.7051)
  line L56 (21.8533, -40.7381) -> (13.3536, -44.2588)
  line L57 (14.5823, -23.1844) -> (21.8533, -40.7381)
  line L58 (6.0826, -26.7051) -> (14.5823, -23.1844)
  line L59 (29.2742, -35.7796) -> (15.8392, -22.3446)
  line L60 (35.7796, -29.2742) -> (29.2742, -35.7796)
  line L61 (22.3446, -15.8392) -> (35.7796, -29.2742)
  line L62 (15.8392, -22.3446) -> (22.3446, -15.8392)
  line L63 (40.7381, -21.8533) -> (23.1844, -14.5823)
  line L64 (44.2588, -13.3536) -> (40.7381, -21.8533)
  line L65 (26.7051, -6.0826) -> (44.2588, -13.3536)
  line L66 (23.1844, -14.5823) -> (26.7051, -6.0826)
  line L67 (46, -4.6) -> (27, -4.6)
  line L68 (46, 4.6) -> (46, -4.6)
  line L69 (27, 4.6) -> (46, 4.6)
  line L70 (27, -4.6) -> (27, 4.6)
  line L71 (44.2588, 13.3536) -> (26.7051, 6.0826)
  line L72 (40.7381, 21.8533) -> (44.2588, 13.3536)
  line L73 (23.1844, 14.5823) -> (40.7381, 21.8533)
  line L74 (26.7051, 6.0826) -> (23.1844, 14.5823)
  line L75 (35.7796, 29.2742) -> (22.3446, 15.8392)
  line L76 (29.2742, 35.7796) -> (35.7796, 29.2742)
  line L77 (15.8392, 22.3446) -> (29.2742, 35.7796)
  line L78 (22.3446, 15.8392) -> (15.8392, 22.3446)
  line L79 (21.8533, 40.7381) -> (14.5823, 23.1844)
  line L80 (13.3536, 44.2588) -> (21.8533, 40.7381)
  line L81 (6.0826, 26.7051) -> (13.3536, 44.2588)
  line L82 (14.5823, 23.1844) -> (6.0826, 26.7051)
  line L83 (4.6, 46) -> (4.6, 27)
  line L84 (-4.6, 46) -> (4.6, 46)
  line L85 (-4.6, 27) -> (-4.6, 46)
  line L86 (4.6, 27) -> (-4.6, 27)
  line L87 (-13.3536, 44.2588) -> (-6.0826, 26.7051)
  line L88 (-21.8533, 40.7381) -> (-13.3536, 44.2588)
  line L89 (-14.5823, 23.1844) -> (-21.8533, 40.7381)
  line L90 (-6.0826, 26.7051) -> (-14.5823, 23.1844)
  line L91 (-29.2742, 35.7796) -> (-15.8392, 22.3446)
  line L92 (-35.7796, 29.2742) -> (-29.2742, 35.7796)
  line L93 (-22.3446, 15.8392) -> (-35.7796, 29.2742)
  line L94 (-15.8392, 22.3446) -> (-22.3446, 15.8392)
  line L95 (-40.7381, 21.8533) -> (-23.1844, 14.5823)
  line L96 (-44.2588, 13.3536) -> (-40.7381, 21.8533)
  line L97 (-26.7051, 6.0826) -> (-44.2588, 13.3536)
  line L98 (-23.1844, 14.5823) -> (-26.7051, 6.0826)
  line L99 (-46, 4.6) -> (-27, 4.6)
  line L100 (-46, -4.6) -> (-46, 4.6)
  line L101 (-27, -4.6) -> (-46, -4.6)
  line L102 (-27, 4.6) -> (-27, -4.6)
  line L103 (-44.2588, -13.3536) -> (-26.7051, -6.0826)
  line L104 (-40.7381, -21.8533) -> (-44.2588, -13.3536)
  line L105 (-23.1844, -14.5823) -> (-40.7381, -21.8533)
  line L106 (-26.7051, -6.0826) -> (-23.1844, -14.5823)
  line L107 (-35.7796, -29.2742) -> (-22.3446, -15.8392)
  line L108 (-29.2742, -35.7796) -> (-35.7796, -29.2742)
  line L109 (-15.8392, -22.3446) -> (-29.2742, -35.7796)
  line L110 (-22.3446, -15.8392) -> (-15.8392, -22.3446)
  line L111 (-21.8533, -40.7381) -> (-14.5823, -23.1844)
  line L112 (-13.3536, -44.2588) -> (-21.8533, -40.7381)
  line L113 (-6.0826, -26.7051) -> (-13.3536, -44.2588)
  line L114 (-14.5823, -23.1844) -> (-6.0826, -26.7051)
  point P0 (0, -36.5)
  dimension "d45" = 9.2
  dimension "d46" = 19
  dimension "d48" = 360
  constraint coincident A0.centre A1.centre
  constraint perpendicular L25 L48
  constraint horizontal L49
  constraint perpendicular L49 L50
  constraint parallel L49 L51
  constraint parallel L50 L52
  constraint coincident L53 P0
  constraint coincident L54 P0
  constraint coincident L48 P0
  measures "d45" distance of L50.end L51.end
  measures "d46" distance of L49.end L50.end
extrude "Extrude11" cut sketch "Sketch7" against normal blind 2.5 contours A79 L47 A80 L81 | A2 L0 A3 L83 | A77 L45 A78 L79 | A4 L2 A5 L85 | A74 L44 A75 L77 | A7 L3 A8 L87 | A72 L42 A73 L75 | A9 L5 A10 L89 | A69 L41 A70 L73 | A12 L6 A13 L91 | A67 L39 A68 L71 | A14 L8 A15 L93 | A64 L38 A65 L69 | A17 L9 A18 L95 | A62 L36 A63 L67 | A19 L11 A20 L97 | A59 L35 A60 L65 | A22 L12 A23 L99 | A57 L33 A58 L63 | A24 L14 A25 L101 | A54 L32 A55 L61 | A27 L15 A28 L103 | A52 L30 A53 L59 | A29 L17 A30 L105 | A49 L29 A50 L57 | A32 L18 A33 L107 | A47 L27 A48 L55 | A34 L20 A35 L109 | A44 L26 A45 L50 | A37 L21 A38 L111 | A42 L24 A43 L52 | A39 L23 A40 L113
